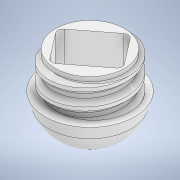
# Autodesk Inventor part: SmartEgg Shell
Saved by Autodesk Inventor 2020 (Build 240168000, 168)
## iProperties
Created: 2019-11-26
Part Number: SmartEgg Shell
Material: Generic
Document SubType Name: Modeling
Designer: Andrew
Density: 1 g/cm^3
Appearance: White
d0: 1.000 ul
d17: 1.000 ul
d18: 25.000 mm
d19: 50.000 mm
d20: 1.000 mm
d21: 17.000 mm
d22: 5.000 mm
d23: 2.000 mm
d24: 12.500 mm
d25: 0.250 mm
d26: 20.000 mm
d27: 3.000 mm
d28: 2.000 mm
d30: 1.000 mm
d32: 0.500 mm
d33: 0.500 mm
d35: 45.00 deg
d36: 0.500 mm
d37: 2.000 mm
d38: 2.000 mm
d41: 9.414 mm
d43: 3.000 ul
d44: 0.00 deg
d50: 9.414 mm
d52: 1.000 ul
d53: 0.00 deg
d61: 2.500 mm
d29: 70.533 mm
d39: 7.000 mm
Thread_Pitch: 4.707 mm
BATT_Width: 24.750 mm
PCB_Width: 22.950 mm
Author: Andrew
Autodesk Inventor part; units mm, degrees
ref_plane "YZ Plane" through (0, 0, 0) normal (1, 0, 0) x (0, 1, 0)
ref_plane "XZ Plane" through (0, 0, 0) normal (0, 1, 0) x (-1, 0, 0)
ref_plane "XY Plane" through (0, 0, 0) normal (0, 0, 1) x (1, 0, 0)
derived "SmartEgg Housing Main.ipt"
sketch "Sketch3" plane through (0, 0, 0) normal (0, 0, 1) x (1, 0, 0)
  line L0 (25.5, 9.7) -> (25.5, -9.55)
  line L1 (26.5, 11.95) -> (26.5, -11.8)
  line L2 (-26.5, -11.8) -> (-26.5, 11.95)
  line L3 (-7.3114, 6.9165) -> (-15.25, -6.8335)
  line L4 (-15.5, -6.7665) -> (-7.5614, 6.9835)
  line L5 (-26.5, 11.95) -> (-7.5614, 11.95)
  line L6 (-7.3114, 11.95) -> (26.5, 11.95)
  line L7 (-25.5, 9.7) -> (7.4386, 9.7)
  line L8 (7.6886, 9.7) -> (25.5, 9.7)
  line L9 (25.5, -9.55) -> (-0.25, -9.55)
  line L10 (-0.5, -9.55) -> (-25.5, -9.55)
  line L11 (26.5, -11.8) -> (-15.25, -11.8)
  line L12 (-15.5, -11.8) -> (-26.5, -11.8)
  line L13 (25.5, 0) -> (25.5, -1.8) construction
  line L14 (-25.5, -1.8) -> (-25.5, 0) construction
  line L15 (-25.5, -3.3) -> (-0.5, -3.3)
  line L16 (-0.5, -3.3) -> (-0.5, -4.3)
  line L17 (-0.5, -4.3) -> (-25.5, -4.3)
  line L18 (-25.5, -9.55) -> (-25.5, -4.3)
  line L19 (-25.5, -3.3) -> (-25.5, 9.7)
  line L20 (-7.4364, 11.95) -> (-7.4364, 6.95) construction
  line L21 (-7.4364, 6.95) -> (-15.375, -6.8) construction
  line L22 (-15.375, -6.8) -> (-15.375, -11.8) construction
  line L23 (-7.5614, 11.95) -> (-7.5614, 10.7)
  line L24 (-7.5614, 10.7) -> (7.4386, 10.7)
  line L25 (7.4386, 10.7) -> (7.4386, 9.7)
  line L26 (7.6886, 9.7) -> (7.6886, 10.95)
  line L27 (7.6886, 10.95) -> (-7.3114, 10.95)
  line L28 (-7.3114, 10.95) -> (-7.3114, 11.95)
  line L29 (-15.5, -11.8) -> (-15.5, -10.55)
  line L30 (-15.5, -10.55) -> (-0.5, -10.55)
  line L31 (-0.5, -10.55) -> (-0.5, -9.55)
  line L32 (-0.25, -9.55) -> (-0.25, -10.8)
  line L33 (-0.25, -10.8) -> (-15.25, -10.8)
  line L34 (-15.25, -10.8) -> (-15.25, -11.8)
  line L35 (-7.5614, 10.7) -> (-7.5614, 6.9835)
  line L36 (-7.3114, 6.9165) -> (-7.3114, 10.95)
  line L37 (-15.5, -10.55) -> (-15.5, -6.7665)
  line L38 (-15.25, -6.8335) -> (-15.25, -10.8)
  line L39 (7.4386, 9.7) -> (7.4386, 6.9835)
  line L40 (7.4386, 6.9835) -> (-0.5, -6.7665)
  line L41 (-0.5, -6.7665) -> (-0.5, -9.55)
  line L42 (-0.25, -9.55) -> (-0.25, -6.8335)
  line L43 (-0.25, -6.8335) -> (7.6886, 6.9165)
  line L44 (7.6886, 6.9165) -> (7.6886, 9.7)
  line L45 (-0.375, -11.8) -> (-0.375, -6.8) construction
  line L46 (-0.375, -6.8) -> (7.5636, 6.95) construction
  line L47 (7.5636, 6.95) -> (7.5636, 11.95) construction
  line L48 (11.5, -9.55) -> (16.5, -9.55)
  line L49 (16.5, -9.55) -> (14, -7.05)
  line L50 (14, -7.05) -> (11.5, -7.05)
  line L51 (11.5, -7.05) -> (11.5, -9.55)
  point P0 (0, 0)
derived "SmartEgg Housing Cap.ipt"
sketch "Housing Largest Area" plane through (0, -10.6204, -14.0095) normal (0, 0.7948428, -0.6068154) x (0, 0.6068154, 0.7948428)
  line L0 (30.7511, 26.5) -> (29.3995, 26.5)
  line L1 (17.6255, 26.5) -> (17.6255, -26.5)
  line L2 (17.6255, -26.5) -> (35.2511, -26.5)
  line L3 (35.2511, -26.5) -> (35.2511, 22)
  line L4 (10.4196, -26.5) -> (24.8315, -26.5) construction
  line L5 (24.8315, 26.5) -> (10.4196, 26.5) construction
  line L6 (12.0637, 20.5) -> (10.4158, 20.5) construction
  line L7 (10.4158, 20.5) -> (10.4158, 24.5) construction
  ellipse E0 centre (8.7678, 24.5) end of major axis (10.4158, 24.5) minor radius 1 (10.4158, 24.5) -> (8.7678, 25.5) ccw construction
  line L8 (8.7678, 25.5) -> (2.3515, 25.5) construction
  line L9 (2.3515, 25.5) -> (2.3515, 16.1435) construction
  line L10 (2.3515, -0.25) -> (1, -0.25) construction
  line L11 (1, -0.25) -> (1, -15.25) construction
  line L12 (1, -15.25) -> (0, -15.25) construction
  line L13 (0, -15.25) -> (0, 26.5) construction
  line L14 (17.0488, 25.5) -> (14.5356, 25.5) construction
  line L15 (14.5356, 25.5) -> (14.5356, 22.4142) construction
  ellipse E1 centre (12.8877, 22.4142) end of major axis (14.5356, 22.4142) minor radius 1 (14.053, 21.7071) -> (14.5356, 22.4142) ccw construction
  line L16 (14.053, 21.7071) -> (12.0637, 20.5) construction
  line L17 (35.2511, 26.5) -> (35.2511, -7.3114) construction
  line L18 (35.2511, -7.3114) -> (34.2511, -7.3114) construction
  line L19 (34.2511, -7.3114) -> (34.2511, 7.6886) construction
  line L20 (34.2511, 7.6886) -> (32.8995, 7.6886) construction
  line L21 (32.8995, 7.6886) -> (32.8995, 25.5) construction
  arc A0 (35.2511, 22) -> (30.7511, 26.5) centre (30.7511, 22) ccw
  arc A1 (32.8995, 22) -> (29.3995, 25.5) centre (29.3995, 22) ccw
  line L22 (32.8995, 22) -> (35.2511, 22)
  line L23 (29.3995, 25.5) -> (29.3995, 26.5)
  line L24 (29.3995, 26.5) -> (17.6255, 26.5)
  line L25 (2.3515, 16.1435) -> (4.5726, 14.7957)
  line L26 (4.5726, 14.7957) -> (4.5726, 11.5)
  line L27 (4.5726, 11.5) -> (2.3515, 11.5)
  line L28 (2.3515, 11.5) -> (2.3515, -0.25)
  line L29 (0, 26.5) -> (17.0488, 26.5)
  line L30 (17.0488, 26.5) -> (17.0488, 25.5)
  line L31 (32.8995, 25.5) -> (21.9926, 25.5)
  line L32 (21.9926, 25.5) -> (21.9926, 26.5)
  line L33 (21.9926, 26.5) -> (35.2511, 26.5)
  point P0 (17.58, 0)
  point P1 (17.6255, 0)
sketch "ESP32 Feather" plane through (0, 0, 0) normal (0, 0, 1) x (1, 0, 0)
  line L0 (-25.5, 0) -> (25.5, 0)
  line L1 (25.5, 0) -> (25.5, -1.8)
  line L2 (25.5, -1.8) -> (-25.5, -1.8)
  line L3 (-25.5, -1.8) -> (-25.5, 0)
  line L4 (0, 0) -> (-25.5, 0)
  line L5 (-25.5, 0) -> (-25.5, 0.75)
  line L6 (-25.5, 0.75) -> (0, 0.75)
  line L7 (0, 0.75) -> (0, 0)
  line L8 (-0.9, 0.75) -> (-18.55, 0.75)
  line L9 (-18.55, 0.75) -> (-18.55, 3.1)
  line L10 (-18.55, 3.1) -> (-0.9, 3.1)
  line L11 (-0.9, 3.1) -> (-0.9, 0.75)
  line L12 (10, 0) -> (18, 0)
  line L13 (18, 0) -> (18, 5.5)
  line L14 (18, 5.5) -> (10, 5.5)
  line L15 (10, 5.5) -> (10, 0)
  line L16 (25.6, 0) -> (19.95, 0)
  line L17 (19.95, 0) -> (19.95, 2.45)
  line L18 (19.95, 2.45) -> (25.6, 2.45)
  line L19 (25.6, 2.45) -> (25.6, 0)
  point P0 (0, 0)
  point P1 (0, 0)
  point P2 (-18.55, 0.75)
  point P3 (18, 0)
  point P4 (19.95, 0)
sketch "Shell Sketch" plane through (0, -10.6204, -14.0095) normal (0, 0.7948428, -0.6068154) x (0, 0.6068154, 0.7948428)
  arc A0 (41.0761, -18.875) -> (29.7061, 33.6321) centre (-5.8251, -1.5465) ccw
  arc A1 (17.6255, -35.2107) -> (30.1255, -31.8614) centre (17.6255, -10.2107) ccw construction
  line L0 (17.6255, -35.2107) -> (17.6255, -31.8614) construction
  line L1 (17.6255, 9) -> (37.2511, 9)
  line L2 (17.6255, 26.5) -> (17.6255, -26.5) construction
  line L3 (35.2511, -26.5) -> (35.9855, -27.1787) construction
  arc A2 (29.7061, 33.6321) -> (17.6255, 38.6714) centre (17.6255, 21.6714) ccw
  line L4 (17.6255, 38.6714) -> (17.6255, 35.8135)
  line L5 (17.6255, 35.8135) -> (22.6255, 35.8135)
  arc A3 (28.2849, 32.225) -> (22.6255, 35.8135) centre (17.6255, 21.6714) ccw
  arc A4 (39.0833, 15.4017) -> (28.2849, 32.225) centre (-5.8251, -1.5465) ccw
  arc A5 (35.2511, 22) -> (30.7511, 26.5) centre (30.7511, 22) ccw construction
  line L6 (37.2511, 9) -> (37.2511, -11.8614)
  line L7 (37.2511, -11.8614) -> (43.0994, -11.8614)
  line L8 (40.2511, 9) -> (40.2511, -11.6114)
  line L9 (40.2511, -11.6114) -> (43.1514, -11.6114)
  line L10 (17.6255, -31.8614) -> (30.1255, -31.8614)
  arc A6 (30.1255, -31.8614) -> (41.0761, -18.875) centre (17.6255, -10.2107) ccw
  line L11 (17.6255, -31.8614) -> (17.6255, 9)
  line L12 (35.2511, -26.5) -> (35.2511, 22) construction
  line L13 (20.9175, 10) -> (17.58, 10) construction
  arc A7 (40.2511, 9) -> (39.0833, 15.4017) centre (22.1205, 9) ccw
  arc A8 (39.2001, -18.1818) -> (40.5683, -13.8614) centre (-5.8251, -1.5465) ccw
  arc A9 (37.2511, -22.204) -> (39.2001, -18.1818) centre (17.6255, -10.2107) ccw
  line L14 (40.5683, -13.8614) -> (37.2511, -13.8614)
  line L15 (37.2511, -13.8614) -> (37.2511, -22.204)
  point P0 (17.58, 0)
  point P1 (40.2511, 11.9068)
  dimension "d18" = 25
  dimension "d19" = 50
  dimension "d20" = 1
  dimension "d21" = 17
  dimension "d22" = 5
  dimension "d23" = 2
  dimension "d24" = 12.5
  dimension "d25" = 0.25
  dimension "d26" = 20
  dimension "d27" = 3
  dimension "d28" = 2
  dimension "d29" = 70.5327
  dimension "d30" = 1
  dimension "d75" = 2
  dimension "d76" = 2
  dimension "d77" = 2
  constraints: 26 end point, 23 point on circle, 9 centre point, 7 line through centre, 7 tangent, 6 perpendicular, 5 vertical, 4 collinear, 4 concentric, 2 horizontal, 2 point on line, 1 coincident
  measures "d18" radius of A1
  measures "d19" radius of A0
  measures "d20" distance of L3.start L3.end
  measures "d21" radius of A2
  measures "d22" distance of L4.end L5.end
  measures "d23" radial gap between concentric circles of A0 A4
  measures "d24" distance of L0.end L10.end
  measures "d25" distance between parallel lines of L7 L9
  measures "d26" distance between parallel lines of L10 L7
  measures "d27" distance between parallel lines of L8 L6
  measures "d28" distance between parallel lines of L12 L6
  measures "d29" distance from line of L10 L4.start
  measures "d30" distance between parallel lines of L1 L13
  measures "d75" radial gap between concentric circles of A0 A8
  measures "d76" distance between parallel lines of L12 L15
  measures "d77" distance between parallel lines of L14 L7
sketch "Thread Sketch" plane through (0, -10.6204, -14.0095) normal (0, 0.7948428, -0.6068154) x (0, 0.6068154, 0.7948428)
  line L0 (37.2511, 9) -> (37.2511, -11.8614) construction
  line L1 (40.2511, 9) -> (40.2511, -11.6114) construction
  line L2 (37.2511, 9) -> (39.7511, 6.5)
  line L3 (39.7511, 6.5) -> (39.7511, 4.5)
  line L4 (39.7511, 4.5) -> (37.2511, 2)
  line L5 (37.2511, 2) -> (37.2511, 9)
  line L6 (40.2511, 4.2929) -> (37.7511, 1.7929)
  line L7 (37.7511, 1.7929) -> (37.7511, -0.2071)
  line L8 (37.7511, -0.2071) -> (40.2511, -2.7071)
  line L9 (40.2511, -2.7071) -> (40.2511, 4.2929)
  line L10 (39.7511, 5.5) -> (37.2511, 5.5) construction
  line L11 (37.7511, 0.7929) -> (40.2511, 0.7929) construction
  point P0 (17.58, 0)
  dimension "d32" = 0.5
  dimension "d33" = 0.5
  dimension "d35" = 45
  dimension "d36" = 0.5
  dimension "d37" = 2
  dimension "d38" = 2
  dimension "d39" = 7
  dimension "Thread_Pitch" = 4.7071
  constraints: 20 end point, 4 midpoint, 3 parallel, 2 horizontal, 2 point on line, 2 other
  measures "d32" distance between parallel lines of L1 L3
  measures "d33" distance between parallel lines of L0 L7
  measures "d35" angle of L0 L4
  measures "d36" distance between parallel lines of L6 L4
  measures "d37" distance of L2.end L3.end
  measures "d38" distance of L6.end L7.end
  measures "d39" distance of L4.end L0.start
  measures "Thread_Pitch" distance between parallel lines of L11 L10
revolve "Revolution1" add sketch "Shell Sketch" angle 360 about axis through (-31.8614, 0.075, 0) along (1, 0, 0) contours A6 L10 L11 L1 L6 L7 A0
coil "Coil1" sketch "Thread Sketch" operation add axis through (-31.8614, 0.075, 0) along (-1, 0, 0) pitch 9.4142 turns 3 hand right separate body contours L2 L3 L4 L5
coil "Coil2" sketch "Thread Sketch" operation add axis through (-31.8614, 0.075, 0) along (1, 0, 0) pitch 9.4142 turns 1 hand right bodies 2 contours L2 L3 L4 L5
sketch "Thread Mask" plane through (0, -10.6204, -14.0095) normal (0, 0.7948428, -0.6068154) x (0, 0.6068154, 0.7948428)
  line L0 (40.2511, 6.5) -> (37.2511, 6.5)
  line L1 (37.2511, 6.5) -> (37.2511, -11.8614)
  line L2 (37.2511, -11.8614) -> (40.2511, -11.8614)
  line L3 (40.2511, -11.8614) -> (40.2511, 6.5)
  line L4 (37.2511, 9) -> (37.2511, -11.8614) construction
  line L5 (40.2511, 9) -> (40.2511, -11.6114) construction
  point P0 (17.58, 0)
  dimension "d61" = 2.5
  constraints: 8 end point, 2 parallel, 1 collinear, 1 horizontal, 1 perpendicular
  measures "d61" distance from line of L4.start L0
revolve "Revolution4" cut sketch "Thread Mask" angle 360 about axis through (-31.8614, 0.075, 0) along (1, 0, 0) keep common part bodies 2
combine bodies "Combine1" operation type add bodies to combine 1 2
sketch "Sketch10" plane through (9, 0.075, 0) normal (1, 0, 0) x (0, 0, -1)
  line L0 (-12.125, -12.125) -> (12.125, -12.125)
  line L1 (15.125, -9.125) -> (15.125, 9.125)
  line L2 (12.125, 12.125) -> (-12.125, 12.125)
  line L3 (-15.125, 9.125) -> (-15.125, -9.125)
  line L4 (-15.125, 0) -> (15.125, 0) construction
  arc A0 (-12.125, 12.125) -> (-15.125, 9.125) centre (-12.125, 9.125) ccw
  arc A1 (15.125, 9.125) -> (12.125, 12.125) centre (12.125, 9.125) ccw
  arc A2 (12.125, -12.125) -> (15.125, -9.125) centre (12.125, -9.125) ccw
  arc A3 (-15.125, -9.125) -> (-12.125, -12.125) centre (-12.125, -9.125) ccw
  point P0 (0, -0.075)
  point P1 (15.125, 12.125)
  point P2 (-15.125, 12.125)
  point P3 (0, -11.875)
  point P4 (0, -11.875)
  point P5 (0, -11.875)
  point P6 (0, 11.875)
  point P7 (0, 11.875)
  point P8 (0, 11.875)
  point P9 (0, 0)
  point P10 (0, 0)
  point P11 (0, 0)
  point P12 (0, 0)
  dimension "d64" = 0.25
  dimension "d65" = 30.25
  dimension "d66" = 3
  constraints: 10 end point, 8 point on circle, 8 tangent, 4 centre point, 4 point on line, 3 equal radius, 3 midpoint, 2 parallel, 1 coincident, 1 horizontal, 1 perpendicular
  measures "d64" distance from line of L0 point (0, -11.875)
  measures "d65" distance of point (15.125, 12.125) point (-15.125, 12.125)
  measures "d66" radius of A0
sketch "Sketch11" plane through (0, 0, 0) normal (0, 0, 1) x (1, 0, 0)
  line L0 (9, 19.7005) -> (9, -19.5505) projected
  line L1 (9, 0.075) -> (-26.5, 0.075)
  line L2 (-26.5, -11.8) -> (-26.5, 11.95) construction
  point P0 (0, 0)
  dimension "d67" = 35.5
  constraints: 2 end point, 2 midpoint, 1 horizontal
  measures "d67" distance of L1.start L1.end
extrude "Extrusion1" cut sketch "Sketch10" against normal blind 35.5 bodies 1
sketch "Vent Lookup" plane through (0, -10.6204, -14.0095) normal (0, 0.7948428, -0.6068154) x (0, 0.6068154, 0.7948428)
  arc A0 (41.0761, -18.875) -> (29.7061, 33.6321) centre (-5.8251, -1.5465) ccw projected
  line L0 (40.8046, 16.5) -> (17.6255, 7.5293)
  line L1 (17.6255, 26.5) -> (17.6255, -26.5) construction
  line L2 (20.9175, 10) -> (17.58, 10) construction
  point P0 (17.58, 0)
  dimension "d71" = 6.5
  constraints: 2 end point, 1 line through centre, 1 point on circle, 1 point on line
  measures "d71" distance from line of L2 L0.start
ref_plane "Vent Plane" through (16.5, 14.1404, 18.4237) normal (-0.3609294, -0.5659119, -0.7412649) x (0.8431188, -0.5377274, 0)
sketch "Sketch13" plane through (-11.8614, 0.075, 0) normal (1, 0, 0) x (0, 0, -1)
  circle A0 centre (0, -0.075) radius 24.75 construction
  dimension "d72" = 49.5
  constraints: 1 centre point, 1 coincident, 1 other
  measures "d72" diameter of A0
emboss "Emboss1" [suppressed]
sketch "Sketch14" plane through (-26.5, 0.075, 0) normal (1, 0, 0) x (0, 0, -1)
  line L0 (-18.1797, 8.0579) -> (18.1797, 8.0579) construction
  line L1 (18.1797, 8.0579) -> (18.1797, -8.2079) construction
  line L2 (18.1797, -8.2079) -> (-18.1797, -8.2079) construction
  line L3 (-18.1797, -8.2079) -> (-18.1797, 8.0579) construction
  line L4 (-7.1317, 7.006) -> (-5.8482, 7.006)
  line L5 (-5.8482, 7.006) -> (-4.1712, 4.5461)
  line L6 (-4.1712, 4.5461) -> (-4.1712, 7.006)
  line L7 (-4.1712, 7.006) -> (-2.8749, 7.006)
  line L8 (-2.8749, 7.006) -> (-2.8749, 2.561)
  line L9 (-2.8749, 2.561) -> (-4.1712, 2.561)
  line L10 (-4.1712, 2.561) -> (-5.8397, 5.0081)
  line L11 (-5.8397, 5.0081) -> (-5.8397, 2.561)
  line L12 (-5.8397, 2.561) -> (-7.1317, 2.561)
  line L13 (-7.1317, 2.561) -> (-7.1317, 7.006)
  line L14 (0.2781, 4.1696) -> (0.2781, 5.0937)
  line L15 (0.2781, 5.0937) -> (2.4, 5.0937)
  line L16 (2.4, 5.0937) -> (2.4, 3.2028)
  spline S0 degree 2 poles (2.4, 3.2028) (1.7883, 2.7835) (0.8514, 2.484) (0.2096, 2.484) knots 0 0 0 1 2 2 2
  spline S1 degree 2 poles (0.2096, 2.484) (-0.5818, 2.484) (-1.5829, 3.0231) (-2.1305, 4.0926) (-2.1305, 4.7857) knots 0 0 0 1 2 3 3 3
  spline S2 degree 2 poles (-2.1305, 4.7857) (-2.1305, 5.513) (-1.5316, 6.5868) (-0.9497, 6.8691) knots 0 0 0 1 2 2 2
  spline S3 degree 2 poles (-0.9497, 6.8691) (-0.4963, 7.083) (0.2652, 7.083) knots 0 0 0 1 1 1
  spline S4 degree 2 poles (0.2652, 7.083) (1.0054, 7.083) (1.7369, 6.8178) (2.2204, 6.2531) (2.3401, 5.8253) knots 0 0 0 1 2 3 3 3
  line L17 (2.3401, 5.8253) -> (1.0139, 5.5857)
  spline S5 degree 2 poles (1.0139, 5.5857) (0.9326, 5.8381) (0.539, 6.1076) (0.2353, 6.1076) knots 0 0 0 1 2 2 2
  spline S6 degree 2 poles (0.2353, 6.1076) (-0.2139, 6.1076) (-0.753, 5.4787) (-0.753, 4.7985) knots 0 0 0 1 2 2 2
  spline S7 degree 2 poles (-0.753, 4.7985) (-0.753, 4.0798) (-0.2096, 3.4594) (0.2781, 3.4594) knots 0 0 0 1 2 2 2
  spline S8 degree 2 poles (0.2781, 3.4594) (0.5091, 3.4594) (0.9284, 3.5921) (1.1979, 3.7546) knots 0 0 0 1 2 2 2
  line L18 (1.1979, 3.7546) -> (1.1979, 4.1696)
  line L19 (1.1979, 4.1696) -> (0.2781, 4.1696)
  line L20 (6.1734, 4.3793) -> (7.3755, 4.0156)
  spline S9 degree 2 poles (7.3755, 4.0156) (7.2557, 3.5108) (6.7338, 2.8306) (5.9595, 2.484) (5.3648, 2.484) knots 0 0 0 1 2 3 3 3
  spline S10 degree 2 poles (5.3648, 2.484) (4.6375, 2.484) (3.722, 2.9076) (3.0546, 3.9685) (3.0546, 4.7942) knots 0 0 0 1 2 3 3 3
  spline S11 degree 2 poles (3.0546, 4.7942) (3.0546, 5.898) (4.2268, 7.083) (5.3006, 7.083) knots 0 0 0 1 2 2 2
  spline S12 degree 2 poles (5.3006, 7.083) (6.1391, 7.083) (7.0975, 6.4028) (7.3328, 5.7012) knots 0 0 0 1 2 2 2
  line L21 (7.3328, 5.7012) -> (6.1178, 5.4317)
  spline S13 degree 2 poles (6.1178, 5.4317) (6.0536, 5.6328) (5.9851, 5.7269) knots 0 0 0 1 1 1
  spline S14 degree 2 poles (5.9851, 5.7269) (5.8696, 5.8852) (5.5359, 6.0563) (5.3306, 6.0563) knots 0 0 0 1 2 2 2
  spline S15 degree 2 poles (5.3306, 6.0563) (4.8685, 6.0563) (4.6204, 5.6798) knots 0 0 0 1 1 1
  spline S16 degree 2 poles (4.6204, 5.6798) (4.4322, 5.4017) (4.4322, 4.8028) knots 0 0 0 1 1 1
  spline S17 degree 2 poles (4.4322, 4.8028) (4.4322, 4.0627) (4.8814, 3.5151) (5.2878, 3.5151) knots 0 0 0 1 2 2 2
  spline S18 degree 2 poles (5.2878, 3.5151) (5.6814, 3.5151) (6.0835, 3.9557) (6.1734, 4.3793) knots 0 0 0 1 2 2 2
  line L22 (-13.3521, -2.788) -> (-9.9595, -2.788)
  line L23 (-9.9595, -2.788) -> (-9.9595, -3.7421)
  line L24 (-9.9595, -3.7421) -> (-11.9703, -3.7421)
  line L25 (-11.9703, -3.7421) -> (-11.9703, -4.5164)
  line L26 (-11.9703, -4.5164) -> (-10.2547, -4.5164)
  line L27 (-10.2547, -4.5164) -> (-10.2547, -5.4148)
  line L28 (-10.2547, -5.4148) -> (-11.9703, -5.4148)
  line L29 (-11.9703, -5.4148) -> (-11.9703, -7.233)
  line L30 (-11.9703, -7.233) -> (-13.3521, -7.233)
  line L31 (-13.3521, -7.233) -> (-13.3521, -2.788)
  line L32 (-6.4814, -6.4972) -> (-8.0429, -6.4972)
  line L33 (-8.0429, -6.4972) -> (-8.2611, -7.233)
  line L34 (-8.2611, -7.233) -> (-9.6643, -7.233)
  line L35 (-9.6643, -7.233) -> (-7.9916, -2.788)
  line L36 (-7.9916, -2.788) -> (-6.49, -2.788)
  line L37 (-6.49, -2.788) -> (-4.8215, -7.233)
  line L38 (-4.8215, -7.233) -> (-6.2589, -7.233)
  line L39 (-6.2589, -7.233) -> (-6.4814, -6.4972)
  line L40 (-6.768, -5.5346) -> (-7.2557, -3.9389)
  line L41 (-7.2557, -3.9389) -> (-7.7435, -5.5346)
  line L42 (-7.7435, -5.5346) -> (-6.768, -5.5346)
  line L43 (-4.3766, -2.788) -> (-1.8054, -2.788)
  spline S19 degree 2 poles (-1.8054, -2.788) (-1.1637, -2.788) (-0.4749, -3.4255) (-0.4749, -3.8961) knots 0 0 0 1 2 2 2
  spline S20 degree 2 poles (-0.4749, -3.8961) (-0.4749, -4.2897) (-0.7187, -4.572) knots 0 0 0 1 1 1
  spline S21 degree 2 poles (-0.7187, -4.572) (-0.8856, -4.7603) (-1.2022, -4.8715) knots 0 0 0 1 1 1
  spline S22 degree 2 poles (-1.2022, -4.8715) (-0.723, -4.987) (-0.2695, -5.5475) (-0.2695, -5.971) knots 0 0 0 1 2 2 2
  spline S23 degree 2 poles (-0.2695, -5.971) (-0.2695, -6.3132) (-0.5904, -6.8651) (-0.8685, -7.0277) knots 0 0 0 1 2 2 2
  spline S24 degree 2 poles (-0.8685, -7.0277) (-1.0439, -7.1261) (-1.3904, -7.1732) knots 0 0 0 1 1 1
  spline S25 degree 2 poles (-1.3904, -7.1732) (-1.8567, -7.233) (-2.0065, -7.233) knots 0 0 0 1 1 1
  line L44 (-2.0065, -7.233) -> (-4.3766, -7.233)
  line L45 (-4.3766, -7.233) -> (-4.3766, -2.788)
  line L46 (-2.9904, -6.279) -> (-2.2931, -6.279)
  spline S26 degree 2 poles (-2.2931, -6.279) (-1.938, -6.279) (-1.6471, -6.0266) (-1.6471, -5.817) knots 0 0 0 1 2 2 2
  spline S27 degree 2 poles (-1.6471, -5.817) (-1.6471, -5.6202) (-1.9337, -5.3806) (-2.2931, -5.3806) knots 0 0 0 1 2 2 2
  line L47 (-2.2931, -5.3806) -> (-2.9904, -5.3806)
  line L48 (-2.9904, -5.3806) -> (-2.9904, -6.279)
  line L49 (-2.9904, -4.5335) -> (-2.3958, -4.5335)
  spline S28 degree 2 poles (-2.3958, -4.5335) (-2.0749, -4.5335) (-1.8225, -4.3111) (-1.8225, -4.1014) knots 0 0 0 1 2 2 2
  spline S29 degree 2 poles (-1.8225, -4.1014) (-1.8225, -3.9089) (-2.0749, -3.6907) (-2.3872, -3.6907) knots 0 0 0 1 2 2 2
  line L50 (-2.3872, -3.6907) -> (-2.9904, -3.6907)
  line L51 (-2.9904, -3.6907) -> (-2.9904, -4.5335)
  line L52 (0.4535, -2.788) -> (1.8268, -2.788)
  line L53 (1.8268, -2.788) -> (1.8268, -6.1378)
  line L54 (1.8268, -6.1378) -> (3.9701, -6.1378)
  line L55 (3.9701, -6.1378) -> (3.9701, -7.233)
  line L56 (3.9701, -7.233) -> (0.4535, -7.233)
  line L57 (0.4535, -7.233) -> (0.4535, -2.788)
  line L58 (7.3328, -6.4972) -> (5.7712, -6.4972)
  line L59 (5.7712, -6.4972) -> (5.553, -7.233)
  line L60 (5.553, -7.233) -> (4.1498, -7.233)
  line L61 (4.1498, -7.233) -> (5.8226, -2.788)
  line L62 (5.8226, -2.788) -> (7.3242, -2.788)
  line L63 (7.3242, -2.788) -> (8.9927, -7.233)
  line L64 (8.9927, -7.233) -> (7.5552, -7.233)
  line L65 (7.5552, -7.233) -> (7.3328, -6.4972)
  line L66 (7.0461, -5.5346) -> (6.5584, -3.9389)
  line L67 (6.5584, -3.9389) -> (6.0707, -5.5346)
  line L68 (6.0707, -5.5346) -> (7.0461, -5.5346)
  line L69 (9.4376, -2.788) -> (12.0088, -2.788)
  spline S30 degree 2 poles (12.0088, -2.788) (12.6505, -2.788) (13.3393, -3.4255) (13.3393, -3.8961) knots 0 0 0 1 2 2 2
  spline S31 degree 2 poles (13.3393, -3.8961) (13.3393, -4.2897) (13.0954, -4.572) knots 0 0 0 1 1 1
  spline S32 degree 2 poles (13.0954, -4.572) (12.9286, -4.7603) (12.612, -4.8715) knots 0 0 0 1 1 1
  spline S33 degree 2 poles (12.612, -4.8715) (13.0911, -4.987) (13.5446, -5.5475) (13.5446, -5.971) knots 0 0 0 1 2 2 2
  spline S34 degree 2 poles (13.5446, -5.971) (13.5446, -6.3132) (13.2238, -6.8651) (12.9457, -7.0277) knots 0 0 0 1 2 2 2
  spline S35 degree 2 poles (12.9457, -7.0277) (12.7703, -7.1261) (12.4238, -7.1732) knots 0 0 0 1 1 1
  spline S36 degree 2 poles (12.4238, -7.1732) (11.9574, -7.233) (11.8077, -7.233) knots 0 0 0 1 1 1
  line L70 (11.8077, -7.233) -> (9.4376, -7.233)
  line L71 (9.4376, -7.233) -> (9.4376, -2.788)
  line L72 (10.8237, -6.279) -> (11.5211, -6.279)
  spline S37 degree 2 poles (11.5211, -6.279) (11.8761, -6.279) (12.1671, -6.0266) (12.1671, -5.817) knots 0 0 0 1 2 2 2
  spline S38 degree 2 poles (12.1671, -5.817) (12.1671, -5.6202) (11.8804, -5.3806) (11.5211, -5.3806) knots 0 0 0 1 2 2 2
  line L73 (11.5211, -5.3806) -> (10.8237, -5.3806)
  line L74 (10.8237, -5.3806) -> (10.8237, -6.279)
  line L75 (10.8237, -4.5335) -> (11.4184, -4.5335)
  spline S39 degree 2 poles (11.4184, -4.5335) (11.7392, -4.5335) (11.9917, -4.3111) (11.9917, -4.1014) knots 0 0 0 1 2 2 2
  spline S40 degree 2 poles (11.9917, -4.1014) (11.9917, -3.9089) (11.7392, -3.6907) (11.4269, -3.6907) knots 0 0 0 1 2 2 2
  line L76 (11.4269, -3.6907) -> (10.8237, -3.6907)
  line L77 (10.8237, -3.6907) -> (10.8237, -4.5335)
  point P0 (0, -0.075)
  point P1 (-18.1797, -0.075)
  point P2 (0, -8.2079)
  constraints: 2 midpoint, 1 horizontal alignment, 1 vertical alignment, 2 other
emboss "Emboss2" sketch "Sketch14" operation cut depth 1 direction (-1, 0, 0)
ref_plane "Work Plane2" through (0, -10.6204, -14.0095) normal (0, 0.7948428, -0.6068154) x (0, 0.6068154, 0.7948428)
equation "\"d38\" = d37"
equation "\"d41\" = 2 * Thread_Pitch"
equation "\"d50\" = 2 * Thread_Pitch"
equation "\"d68\" = d67"
body "Solid1"
body "Solid3"
